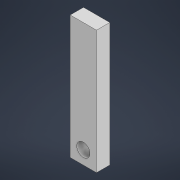
# Autodesk Inventor part: Elbow_Cube_Holder_TestFit_V2
Saved by Autodesk Inventor 2022 (Build 260153000, 153)
## iProperties
Created: 2023-05-10
Part Number: Elbow_Cube_Holder_TestFit_V2
Material: Generic
Document SubType Name: Modeling
Designer: Karl Spiteri
Density: 1 g/cm^3
Appearance: Default
Author: Karl Spiteri
Autodesk Inventor part; units mm, degrees
ref_plane "YZ Plane" through (0, 0, 0) normal (1, 0, 0) x (0, 1, 0)
ref_plane "XZ Plane" through (0, 0, 0) normal (0, 1, 0) x (-1, 0, 0)
ref_plane "XY Plane" through (0, 0, 0) normal (0, 0, 1) x (1, 0, 0)
sketch "Sketch2" plane through (0, 0, 0) normal (0, 0, 1) x (1, 0, 0)
  line L0 (0, 0) -> (-9.9, 0)
  line L1 (-4.95, 0) -> (-4.95, 2.5)
  line L2 (-4.95, 0) -> (-2.45, 0) construction
  circle A0 centre (-4.95, 5) radius 2.5
  line L3 (-4.95, 7.5) -> (32.05, 7.5) construction
  line L4 (0, 44.5) -> (0, 0)
  line L5 (0, 0) -> (-9.9, 0)
  line L6 (-9.9, 0) -> (-9.9, 44.5)
  line L7 (0, 45.5) -> (0, 0)
  line L8 (0, 0) -> (-9.9, 0)
  line L9 (-9.9, 0) -> (-9.9, 45.5)
  line L10 (-4.95, 7.5) -> (66.05, 7.5) construction
  line L11 (0, 0) -> (-9.9, 0)
  line L12 (-9.9, 0) -> (-9.9, 46.5)
  line L13 (-9.9, 46.5) -> (0, 46.5)
  line L14 (0, 46.5) -> (0, 0)
  dimension "d35" = 5
  dimension "d33" = 2.5
  dimension "d34" = 90
  dimension "d46" = 46.5
  constraints: 30 end point, 5 horizontal, 4 parallel, 2 perpendicular, 1 midpoint, 1 point on line, 1 vertical, 1 vertical alignment, 2 other
  measures "d33" distance of L1.start L1.end
  measures "d34" angle of L2 L1
  measures "d46" distance of L11.end L12.end
extrude "Extrusion6" add sketch "Sketch2" along normal blind 5
body "Solid5"
